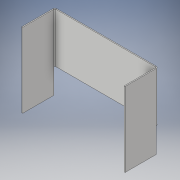
# Autodesk Inventor part: Chute(2)
Saved by Autodesk Inventor 2017 (Build 210142000, 142)
## iProperties
Created: 2017-01-21
Part Number: Chute(2)
Material: Generic
Document SubType Name: Sheet Metal
Designer: kingb
Density: 1 g/cm^3
Sheet Metal Rule: Default
Appearance: Default
Author: kingb
Autodesk Inventor part; units mm, degrees
ref_plane "YZ Plane" through (0, 0, 0) normal (1, 0, 0) x (0, 1, 0)
ref_plane "XZ Plane" through (0, 0, 0) normal (0, 1, 0) x (-1, 0, 0)
ref_plane "XY Plane" through (0, 0, 0) normal (0, 0, 1) x (1, 0, 0)
sketch "Sketch1" plane through (0, 0, 0) normal (0, 0, 1) x (1, 0, 0)
  line L0 (0, 0) -> (317.5, 0)
  line L1 (317.5, 0) -> (317.5, 152.4)
  line L2 (317.5, 152.4) -> (0, 152.4)
  line L3 (0, 152.4) -> (0, 0)
  dimension "d0" = 317.5
  dimension "d1" = 152.4
  measures "d0" distance of L2.end L1.end
  measures "d1" distance of L1.end L0.end
extrude "Plate1" add sketch "Sketch1" along normal blind 3.048
sketch "Sketch2" plane through (3.048, 0, 0) normal (-1, 0, 0) x (0, -1, 0)
  line L0 (-152.4, 0) -> (0, 0)
  line L1 (0, 0) -> (0, 101.6)
  line L2 (0, 101.6) -> (-152.4, 101.6)
  line L3 (-152.4, 101.6) -> (-152.4, 0)
  constraints: 6 end point, 1 horizontal, 1 perpendicular, 1 vertical
edge flange "Flange1" height 101.6 angle 90 thickness 3.048 bend radius 3.048 thickness toward (-1, 0, 0) relief tear relief width 3.048 relief depth 1.524 corner gap 3.048 corner form 0 edges at (0, 76.2, 3.048) (317.5, 76.2, 3.048) wall of the first edge with corners at (3.048, 152.4, 0) (3.048, 0, 0) (3.048, 0, 101.6) (3.048, 152.4, 101.6)
bend "Bend1"
corner "Corner1"
sketch "Sketch3" plane through (0, 0, 101.6) normal (0, -1, 0) x (1, 0, 0)
  line L0 (0, -95.504) -> (3.048, -95.504) projected
  line L1 (3.048, 0) -> (3.048, -95.504) projected
  line L2 (3.048, 0) -> (0, 0) projected
  line L3 (0, 0) -> (0, -95.504) projected
  line L4 (314.452, -95.504) -> (317.5, -95.504) projected
  line L5 (317.5, -95.504) -> (317.5, 0) projected
  line L6 (314.452, 0) -> (317.5, 0) projected
  line L7 (314.452, 0) -> (314.452, -95.504) projected
  point P0 (0, -101.6)
extrude "Extrusion1" add sketch "Sketch3" along normal blind 76.2
equation "\"d3\" = BendReliefWidth"
equation "\"d4\" = BendReliefDepth"
equation "\"d5\" = MinimumRemnant"
equation "\"d6\" = BendRadius"
equation "\"d9\" = BendRadius"
equation "\"d10\" = CornerReliefSize"
equation "\"d11\" = GapSize"
equation "\"d12\" = JacobiRadiusSize"
equation "\"BendRadius\" = Thickness"
equation "\"BendReliefWidth\" = Thickness"
equation "\"BendReliefDepth\" = 0.5 * Thickness"
equation "\"CornerReliefSize\" = 4 * Thickness"
equation "\"MinimumRemnant\" = 2 * Thickness"
equation "\"TransitionRadius\" = BendRadius"
equation "\"JacobiRadiusSize\" = BendRadius"
equation "\"GapSize\" = Thickness"
equation "\"d2\" = BendRadius"
equation "\"Thickness\" = 3.048"
body "Solid1"
